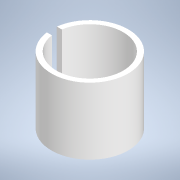
# Autodesk Inventor part: Part1
Saved by Autodesk Inventor 2021 (Build 250183000, 183)
## iProperties
Created: 2021-05-21
Part Number: Part1
Material: PC/ABS Plastic
Document SubType Name: Modeling
Designer: sami8
Density: 0.357273 g/cm^3
Appearance: Smooth - White
Author: sami8
Autodesk Inventor part; units mm, degrees
ref_plane "YZ Plane" through (0, 0, 0) normal (1, 0, 0) x (0, 1, 0)
ref_plane "XZ Plane" through (0, 0, 0) normal (0, 1, 0) x (-1, 0, 0)
ref_plane "XY Plane" through (0, 0, 0) normal (0, 0, 1) x (1, 0, 0)
sketch "Sketch1" plane through (0, 0, 0) normal (0, 1, 0) x (-1, 0, 0)
  circle A0 centre (0, 0) radius 10
  circle A1 centre (0, 0) radius 11.5
  line L0 (0, 1.5) -> (16, 1.5)
  line L1 (16, 1.5) -> (16, -1.5)
  line L2 (16, -1.5) -> (0, -1.5)
  line L3 (0, -1.5) -> (0, 1.5)
  point P0 (11.4018, -1.5)
  point P1 (9.8869, -1.5)
  point P2 (9.8869, 1.5)
  point P3 (11.4018, 1.5)
  dimension "d0" = 20
  dimension "d1" = 23
  dimension "d2" = 3
  dimension "d3" = 16
  constraints: 8 end point, 3 coincident, 2 centre point, 2 parallel, 1 horizontal, 1 midpoint, 1 perpendicular
  measures "d0" diameter of A0
  measures "d1" diameter of A1
  measures "d2" distance of L0.end L1.end
  measures "d3" distance between parallel lines of L3 L1
extrude "Extrusion1" add sketch "Sketch1" along normal blind 20 contours A0 L2 A1 L0 picked at (10.6678, 2.3922)
body "Solid1"
